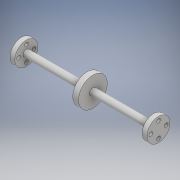
# Autodesk Inventor part: 煞車桿
Saved by Autodesk Inventor 2019 (Build 230136000, 136)
## iProperties
Created: 2020-03-18
Part Number: 煞車桿
Material: 一般
Document SubType Name: Modeling
Designer: 黃柏維
Density: 1 g/cm^3
Appearance: 預設
Author: 黃柏維
Autodesk Inventor part; units mm, degrees
ref_plane "YZ Plane" through (0, 0, 0) normal (1, 0, 0) x (0, 1, 0)
ref_plane "XZ Plane" through (0, 0, 0) normal (0, 1, 0) x (-1, 0, 0)
ref_plane "XY Plane" through (0, 0, 0) normal (0, 0, 1) x (1, 0, 0)
sketch "草圖1" plane through (0, 0, 0) normal (1, 0, 0) x (0, 1, 0)
  circle A0 centre (0, 0) radius 15
  dimension "d0" = 30
  constraints: 1 centre point, 1 coincident
  measures "d0" diameter of A0
extrude "擠出1" add sketch "草圖1" along normal mid plane 6
sketch "草圖2" plane through (3, 0, 0) normal (1, 0, 0) x (0, 0, -1)
  circle A0 centre (0, 0) radius 3.5
  dimension "d3" = 7
  constraints: 1 centre point, 1 coincident
  measures "d3" diameter of A0
extrude "擠出2" add sketch "草圖2" along normal blind 68.5
sketch "草圖3" plane through (-3, 0, 0) normal (-1, 0, 0) x (0, 0, 1)
  circle A0 centre (0, 0) radius 3.5
  dimension "d6" = 7
  constraints: 1 centre point, 1 coincident
  measures "d6" diameter of A0
extrude "擠出3" add sketch "草圖3" along normal blind 68.5
sketch "草圖9" plane through (-71.5, 0, 0) normal (-1, 0, 0) x (0, 0, 1)
  circle A0 centre (0, 0) radius 12
  dimension "d27" = 24
  constraints: 1 centre point, 1 coincident
  measures "d27" diameter of A0
extrude "擠出8" add sketch "草圖9" against normal blind 5
sketch "草圖11" plane through (71.5, 0, 0) normal (1, 0, 0) x (0, 0, -1)
  circle A0 centre (0, 0) radius 12
  dimension "d30" = 24
  constraints: 1 centre point, 1 coincident
  measures "d30" diameter of A0
extrude "擠出9" add sketch "草圖11" against normal blind 5
sketch "草圖12" plane through (71.5, 0, 0) normal (1, 0, 0) x (0, 0, -1)
  circle A0 centre (0, -8) radius 2
  circle A1 centre (8, 0) radius 2
  circle A2 centre (0, 8) radius 2
  circle A3 centre (-8, 0) radius 2
  point P0 (0, 0)
  dimension "d33" = 4
  dimension "d36" = 360
  constraints: 4 centre point, 1 coincident, 9 other
  measures "d33" diameter of A0
extrude "擠出10" cut sketch "草圖12" against normal blind 5
sketch "草圖13" plane through (-71.5, 0, 0) normal (-1, 0, 0) x (0, 0, 1)
  circle A0 centre (0, -8) radius 2
  circle A1 centre (8, 0) radius 2
  circle A2 centre (0, 8) radius 2
  circle A3 centre (-8, 0) radius 2
  point P0 (0, 0)
  dimension "d40" = 4
  dimension "d43" = 360
  constraints: 4 centre point, 1 coincident, 9 other
  measures "d40" diameter of A0
extrude "擠出11" cut sketch "草圖13" against normal blind 5
